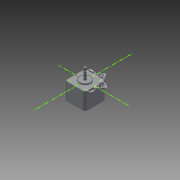
# Autodesk Inventor part: Stepper_Motor
Saved by Autodesk Inventor 2015 (Build 190159000, 159)
## iProperties
Created: 2014-12-21
Part Number: Stepper_Motor
Material: Generic
Document SubType Name: Modeling
Designer: Drew
Density: 1 g/cm^3
Appearance: Default
Author: Drew
Autodesk Inventor part; units mm, degrees
ref_plane "YZ Plane" through (0, 0, 0) normal (1, 0, 0) x (0, 1, 0)
ref_plane "XZ Plane" through (0, 0, 0) normal (0, 1, 0) x (-1, 0, 0)
ref_plane "XY Plane" through (0, 0, 0) normal (0, 0, 1) x (1, 0, 0)
sketch "Sketch1" plane through (0, 0, 0) normal (0, 1, 0) x (-1, 0, 0)
  line L0 (-17.975, -21.15) -> (17.975, -21.15)
  line L1 (21.15, -17.975) -> (21.15, 17.975)
  line L2 (17.975, 21.15) -> (-17.975, 21.15)
  line L3 (-21.15, 17.975) -> (-21.15, -17.975)
  line L4 (-21.15, -21.15) -> (21.15, 21.15) construction
  line L5 (21.15, -21.15) -> (-21.15, 21.15) construction
  line L6 (17.975, 21.15) -> (21.15, 17.975)
  line L7 (-17.975, 21.15) -> (-21.15, 17.975)
  line L8 (-21.15, -17.975) -> (-17.975, -21.15)
  line L9 (17.975, -21.15) -> (21.15, -17.975)
  point P0 (0, 0)
  dimension "d0" = 42.3
  dimension "d1" = 42.3
  dimension "d2" = 3.175
  dimension "d3" = 3.175
  dimension "d4" = 3.175
  dimension "d5" = 3.175
  dimension "d6" = 3.175
  dimension "d7" = 3.175
  dimension "d8" = 3.175
  dimension "d9" = 3.175
  constraints: 20 end point, 8 point on line, 2 midpoint, 2 parallel, 1 horizontal, 1 perpendicular
  measures "d0" distance of L5.start L4.end
  measures "d1" distance of L4.end L5.end
  measures "d2" distance of L2.start L4.end
  measures "d3" distance of L1.end L4.end
  measures "d4" distance of L2.end L5.end
  measures "d5" distance of L3.start L5.end
  measures "d6" distance of L3.end L4.start
  measures "d7" distance of L0.start L4.start
  measures "d8" distance of L0.end L5.start
  measures "d9" distance of L1.start L5.start
extrude "Extrusion1" add sketch "Sketch1" along normal blind 34
sketch "Sketch2" plane through (0, 34, 0) normal (0, 1, 0) x (1, 0, 0)
  circle A0 centre (0, 0) radius 11
  dimension "d12" = 22
  constraints: 1 centre point, 1 coincident
  measures "d12" diameter of A0
extrude "Extrusion2" add sketch "Sketch2" along normal blind 2
sketch "Sketch3" plane through (0, 36, 0) normal (0, 1, 0) x (1, 0, 0)
  circle A0 centre (0, 0) radius 2.5
  dimension "d15" = 5
  constraints: 1 centre point, 1 coincident
  measures "d15" diameter of A0
extrude "Extrusion3" add sketch "Sketch3" along normal blind 22
sketch "Sketch4" plane through (0, 34, 0) normal (0, 1, 0) x (1, 0, 0)
  line L0 (89.125, 0) -> (-55.025, 0)
  line L1 (0, 94.2917) -> (0, -108.2417)
  point P0 (0, 0)
  point P1 (15.5, 15.5)
  point P2 (15.5, -15.5)
  point P3 (-15.5, 15.5)
  point P4 (-15.5, -15.5)
  dimension "d18" = 31
  dimension "d19" = 31
  constraints: 4 end point, 3 symmetric about line, 1 horizontal, 1 vertical
  measures "d18" diameter of point (15.5, 15.5) L0
  measures "d19" diameter of point (15.5, 15.5) L1
equation "\"d1\" = d0"
equation "\"d3\" = d2"
equation "\"d4\" = d2"
equation "\"d5\" = d4"
equation "\"d6\" = d2"
equation "\"d7\" = d6"
equation "\"d8\" = d2"
equation "\"d9\" = d8"
body "Solid1"
